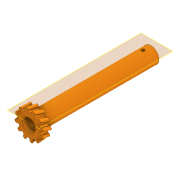
# Autodesk Inventor part: 5th Axis Tube
Saved by Autodesk Inventor 2020 (Build 240168000, 168)
## iProperties
Created: 2021-06-26
Part Number: 5th Axis Tube
Material: Generic
Document SubType Name: Modeling
Designer: Coy
Density: 1 g/cm^3
Appearance: Orange
Author: Coy
Autodesk Inventor part; units mm, degrees
ref_plane "YZ Plane" through (0, 0, 0) normal (1, 0, 0) x (0, 1, 0)
ref_plane "XY Plane" through (0, 0, 0) normal (0, 0, 1) x (1, 0, 0)
sketch "Sketch1" plane through (0, 0, 0) normal (0, 0, 1) x (1, 0, 0)
  circle A0 centre (0, 0) radius 5
  circle A1 centre (0, 0) radius 4
  dimension "d0" = 10
  dimension "d1" = 8
  constraints: 2 centre point, 2 coincident
  measures "d0" diameter of A0
  measures "d1" diameter of A1
extrude "Extrusion1" add sketch "Sketch1" along normal blind 76
ref_plane "Work Plane1" through (0, 0, 71) normal (0, 0, 1) x (1, 0, 0)
sketch "Sketch3" plane through (0, 0, 71) normal (0, 0, 1) x (1, 0, 0)
  circle A0 centre (0, 0) radius 9 construction
  line L0 (0, 0) -> (0, 12.6583) construction
  arc A1 (0.9922, 7.875) -> (-0.9922, 7.875) centre (0, 8) ccw
  line L1 (0.967, 7.675) -> (0.9922, 7.875)
  line L2 (-0.967, 7.675) -> (-0.9922, 7.875)
  arc A2 (-1.7079, 6.582) -> (-0.967, 7.675) centre (-1.9591, 7.55) ccw
  arc A3 (0.967, 7.675) -> (1.7079, 6.582) centre (1.9591, 7.55) ccw
  arc A4 (-4.7701, 4.8462) -> (-4.6749, 6.1632) centre (-5.4716, 5.5589) ccw
  line L3 (-4.6749, 6.1632) -> (-4.7967, 6.3239)
  arc A5 (-3.0783, 7.316) -> (-4.7967, 6.3239) centre (-4, 6.9282) ccw
  line L4 (-3.0001, 7.1302) -> (-3.0783, 7.316)
  arc A6 (-3.0001, 7.1302) -> (-1.8119, 6.5542) centre (-2.0783, 7.518) ccw
  arc A7 (-6.5542, 1.8119) -> (-7.1302, 3.0001) centre (-7.518, 2.0783) ccw
  line L5 (-7.1302, 3.0001) -> (-7.316, 3.0783)
  arc A8 (-6.3239, 4.7967) -> (-7.316, 3.0783) centre (-6.9282, 4) ccw
  line L6 (-6.1632, 4.6749) -> (-6.3239, 4.7967)
  arc A9 (-6.1632, 4.6749) -> (-4.8462, 4.7701) centre (-5.5589, 5.4716) ccw
  arc A10 (-6.582, -1.7079) -> (-7.675, -0.967) centre (-7.55, -1.9591) ccw
  line L7 (-7.675, -0.967) -> (-7.875, -0.9922)
  arc A11 (-7.875, 0.9922) -> (-7.875, -0.9922) centre (-8, 0) ccw
  line L8 (-7.675, 0.967) -> (-7.875, 0.9922)
  arc A12 (-7.675, 0.967) -> (-6.582, 1.7079) centre (-7.55, 1.9591) ccw
  arc A13 (-4.8462, -4.7701) -> (-6.1632, -4.6749) centre (-5.5589, -5.4716) ccw
  line L9 (-6.1632, -4.6749) -> (-6.3239, -4.7967)
  arc A14 (-7.316, -3.0783) -> (-6.3239, -4.7967) centre (-6.9282, -4) ccw
  line L10 (-7.1302, -3.0001) -> (-7.316, -3.0783)
  arc A15 (-7.1302, -3.0001) -> (-6.5542, -1.8119) centre (-7.518, -2.0783) ccw
  arc A16 (-1.8119, -6.5542) -> (-3.0001, -7.1302) centre (-2.0783, -7.518) ccw
  line L11 (-3.0001, -7.1302) -> (-3.0783, -7.316)
  arc A17 (-4.7967, -6.3239) -> (-3.0783, -7.316) centre (-4, -6.9282) ccw
  line L12 (-4.6749, -6.1632) -> (-4.7967, -6.3239)
  arc A18 (-4.6749, -6.1632) -> (-4.7701, -4.8462) centre (-5.4716, -5.5589) ccw
  arc A19 (1.7079, -6.582) -> (0.967, -7.675) centre (1.9591, -7.55) ccw
  line L13 (0.967, -7.675) -> (0.9922, -7.875)
  arc A20 (-0.9922, -7.875) -> (0.9922, -7.875) centre (0, -8) ccw
  line L14 (-0.967, -7.675) -> (-0.9922, -7.875)
  arc A21 (-0.967, -7.675) -> (-1.7079, -6.582) centre (-1.9591, -7.55) ccw
  arc A22 (4.7701, -4.8462) -> (4.6749, -6.1632) centre (5.4716, -5.5589) ccw
  line L15 (4.6749, -6.1632) -> (4.7967, -6.3239)
  arc A23 (3.0783, -7.316) -> (4.7967, -6.3239) centre (4, -6.9282) ccw
  line L16 (3.0001, -7.1302) -> (3.0783, -7.316)
  arc A24 (3.0001, -7.1302) -> (1.8119, -6.5542) centre (2.0783, -7.518) ccw
  arc A25 (6.5542, -1.8119) -> (7.1302, -3.0001) centre (7.518, -2.0783) ccw
  line L17 (7.1302, -3.0001) -> (7.316, -3.0783)
  arc A26 (6.3239, -4.7967) -> (7.316, -3.0783) centre (6.9282, -4) ccw
  line L18 (6.1632, -4.6749) -> (6.3239, -4.7967)
  arc A27 (6.1632, -4.6749) -> (4.8462, -4.7701) centre (5.5589, -5.4716) ccw
  arc A28 (6.582, 1.7079) -> (7.675, 0.967) centre (7.55, 1.9591) ccw
  line L19 (7.675, 0.967) -> (7.875, 0.9922)
  arc A29 (7.875, -0.9922) -> (7.875, 0.9922) centre (8, 0) ccw
  line L20 (7.675, -0.967) -> (7.875, -0.9922)
  arc A30 (7.675, -0.967) -> (6.582, -1.7079) centre (7.55, -1.9591) ccw
  arc A31 (4.8462, 4.7701) -> (6.1632, 4.6749) centre (5.5589, 5.4716) ccw
  line L21 (6.1632, 4.6749) -> (6.3239, 4.7967)
  arc A32 (7.316, 3.0783) -> (6.3239, 4.7967) centre (6.9282, 4) ccw
  line L22 (7.1302, 3.0001) -> (7.316, 3.0783)
  arc A33 (7.1302, 3.0001) -> (6.5542, 1.8119) centre (7.518, 2.0783) ccw
  arc A34 (1.8119, 6.5542) -> (3.0001, 7.1302) centre (2.0783, 7.518) ccw
  line L23 (3.0001, 7.1302) -> (3.0783, 7.316)
  arc A35 (4.7967, 6.3239) -> (3.0783, 7.316) centre (4, 6.9282) ccw
  line L24 (4.6749, 6.1632) -> (4.7967, 6.3239)
  arc A36 (4.6749, 6.1632) -> (4.7701, 4.8462) centre (5.4716, 5.5589) ccw
  arc A37 (-1.7079, 6.582) -> (-1.8119, 6.5542) centre (0, 0) ccw
  arc A38 (1.8119, 6.5542) -> (1.7079, 6.582) centre (0, 0) ccw
  arc A39 (4.8462, 4.7701) -> (4.7701, 4.8462) centre (0, 0) ccw
  arc A40 (6.582, 1.7079) -> (6.5542, 1.8119) centre (0, 0) ccw
  arc A41 (6.5542, -1.8119) -> (6.582, -1.7079) centre (0, 0) ccw
  arc A42 (4.7701, -4.8462) -> (4.8462, -4.7701) centre (0, 0) ccw
  arc A43 (1.7079, -6.582) -> (1.8119, -6.5542) centre (0, 0) ccw
  arc A44 (-1.8119, -6.5542) -> (-1.7079, -6.582) centre (0, 0) ccw
  arc A45 (-4.8462, -4.7701) -> (-4.7701, -4.8462) centre (0, 0) ccw
  arc A46 (-6.582, -1.7079) -> (-6.5542, -1.8119) centre (0, 0) ccw
  arc A47 (-4.7701, 4.8462) -> (-4.8462, 4.7701) centre (0, 0) ccw
  arc A48 (-6.5542, 1.8119) -> (-6.582, 1.7079) centre (0, 0) ccw
  circle A49 centre (0, 0) radius 5 projected
  dimension "d8" = 18
  dimension "d10" = 2
  dimension "d11" = 2
  dimension "d12" = 2
  dimension "d15" = 360
  constraints: 96 point on circle, 50 end point, 49 centre point, 24 line through centre, 5 tangent, 1 coincident, 1 point on line, 1 vertical, 169 other
  measures "d8" diameter of A0
  measures "d10" diameter of A1
  measures "d11" diameter of A2
  measures "d12" diameter of A3
sketch3d "3D Sketch1"
  helix H0 starts at (4.8423, -4.7663, 71) axis through (0, 0, 71) along (0, 0, 1) pitch 166.6667 turns 0.03 hand right
sweep "Sweep1" add profiles "Sketch3" path "3D Sketch1"
sketch "Sketch4" plane through (0, 0, 0) normal (0, 1, 0) x (-1, 0, 0)
  line L0 (5, 0) -> (-5, 0) construction
  line L1 (5, 0) -> (5, 5) construction
  line L2 (5, 0) -> (5, 71) construction
  line L3 (5, 5) -> (5, 5) construction
  line L4 (5, 5) -> (-5, 5) construction
  line L5 (-5, 0) -> (-5, 71) construction
  circle A0 centre (0, 5) radius 1
  point P0 (0, 0)
  dimension "d23" = 5
  dimension "d25" = 2
  dimension "d32" = 5
  constraints: 6 end point, 3 point on line, 2 midpoint, 1 centre point, 1 horizontal
  measures "d23" distance of L0.start L1.end
  measures "d25" diameter of A0
  measures "d32" distance of point (0, 0) A0.centre
extrude "Extrusion3" cut sketch "Sketch4" against normal mid plane 76
ref_plane "Work Plane2" through (0, 0, 2.5) normal (0, 0, -1) x (-1, 0, 0)
sketch "Sketch5" plane through (0, 0, 2.5) normal (0, 0, -1) x (-1, 0, 0)
  circle A0 centre (0, 0) radius 4 projected
  circle A1 centre (0, 0) radius 3.5
  dimension "d29" = 7
  constraints: 1 centre point, 1 coincident
  measures "d29" diameter of A1
extrude "Extrusion4" add sketch "Sketch5" against normal blind 71
ref_plane "Work Plane3" through (0, 5, 0) normal (0, 1, 0) x (-1, 0, 0)
sketch "Sketch6" plane through (0, 5, 0) normal (0, 1, 0) x (-1, 0, 0)
  spline S0 degree 7 poles (1, 5) (1, 5.1216) (0.9828, 5.2432) (0.9483, 5.3627) (0.8964, 5.4779) (0.8272, 5.5863) (0.7407, 5.6851) (0.5413, 5.85) (0.4285, 5.9198) (0.3015, 5.9732) (0.1647, 6.006) (0.0237, 6.0159) (-0.1158, 6.0027) (-0.3809, 5.9346) (-0.5033, 5.8808) (-0.6133, 5.8103) (-0.7093, 5.7265) (-0.7901, 5.6324) (-0.8552, 5.5312) (-0.9587, 5.3112) (-0.9953, 5.1896) (-1.0138, 5.0637) (-1.0138, 4.9363) (-0.9953, 4.8104) (-0.9587, 4.6888) (-0.8585, 4.4757) (-0.7986, 4.381) (-0.7252, 4.2924) (-0.6385, 4.2123) (-0.5394, 4.1433) (-0.429, 4.0879) (-0.1898, 4.0102) (-0.0626, 3.9882) (0.0683, 3.9855) (0.1981, 4.003) (0.322, 4.0395) (0.4355, 4.092) (0.6673, 4.2391) (0.7782, 4.343) (0.8671, 4.4614) (0.9337, 4.5899) (0.9779, 4.7247) (1, 4.8624) (1, 5) knots 0 0 0 0 0 0 0 0 0.148858 0.148858 0.148858 0.148858 0.148858 0.148858 0.287408 0.287408 0.287408 0.287408 0.287408 0.287408 0.425292 0.425292 0.425292 0.425292 0.425292 0.425292 0.575122 0.575122 0.575122 0.575122 0.575122 0.575122 0.704022 0.704022 0.704022 0.704022 0.704022 0.704022 0.83211 0.83211 0.83211 0.83211 0.83211 0.83211 1 1 1 1 1 1 1 1 projected
  point P0 (0, 0)
  constraints: 1 other
extrude "Extrusion5" cut sketch "Sketch6" against normal blind 76
body "Solid1"
